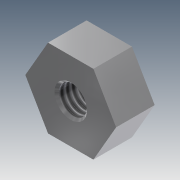
# Autodesk Inventor part: ruka_sroub.-matka
Saved by Autodesk Inventor 2013 (Build 170138000, 138)
## iProperties
Created: 2013-02-16
Part Number: ruka_sroub.-matka
Material: Generic
Document SubType Name: Modeling
Designer: idle-rug
Density: 1 g/cm^3
Author: idle-rug
Autodesk Inventor part; units mm, degrees
ref_plane "YZ Plane" through (0, 0, 0) normal (1, 0, 0) x (0, 1, 0)
ref_plane "XZ Plane" through (0, 0, 0) normal (0, 1, 0) x (-1, 0, 0)
ref_plane "XY Plane" through (0, 0, 0) normal (0, 0, 1) x (1, 0, 0)
sketch "Sketch1" plane through (0, 0, 0) normal (0, 1, 0) x (-1, 0, 0)
  circle A0 centre (0, 0) radius 4
  line L0 (-4, 0) -> (-2, 3.4641)
  line L1 (-2, 3.4641) -> (2, 3.4641)
  line L2 (2, 3.4641) -> (4, 0)
  line L3 (-4, 0) -> (-2, -3.4641)
  line L4 (-2, -3.4641) -> (2, -3.4641)
  line L5 (2, -3.4641) -> (4, 0)
  line L6 (2, 3.4641) -> (-2, 3.4641)
  line L7 (-2, 3.4641) -> (-4, 0)
  line L8 (4, 0) -> (2, 3.4641)
  line L9 (-2, -3.4641) -> (-4, 0)
  line L10 (2, -3.4641) -> (-2, -3.4641)
  line L11 (4, 0) -> (2, -3.4641)
  dimension "d0" = 8
  constraints: 24 end point, 3 equal length, 2 point on line, 1 coincident, 1 horizontal, 10 other
extrude "Extrusion1" add sketch "Sketch1" along normal blind 3.4 contours L5 L4 L3 L0 L1 L2
sketch "Sketch2" plane through (0, 3.4, 0) normal (0, 1, 0) x (1, 0, 0)
  point P0 (0, 0)
hole "Hole1" at (0, 3.4, 0) direction (0, -1, 0) diameter 2.459 depth 3.4 tip angle 118 thread size "M3x0.5" designation "M3" class "6H" standard "GB Metric profile"
chamfer "Chamfer1" distance 0.2 angle 45 1 edges at (0, 3.4, -1.2295)
chamfer "Chamfer2" distance 0.2 angle 45 1 edges at (0, 0, -1.2295)
body "Solid1"
